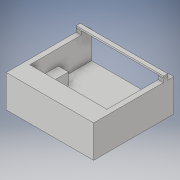
# Autodesk Inventor part: 0 - Ute
Saved by Autodesk Inventor 2019 (Build 230136000, 136)
## iProperties
Created: 2018-07-18
Part Number: 0 - Ute
Material: Generic
Document SubType Name: Modeling
Designer: Samuel
Density: 1 g/cm^3
Appearance: Default
Author: Samuel
Autodesk Inventor part; units mm, degrees
ref_plane "YZ Plane" through (0, 0, 0) normal (1, 0, 0) x (0, 1, 0)
ref_plane "XZ Plane" through (0, 0, 0) normal (0, 1, 0) x (-1, 0, 0)
ref_plane "XY Plane" through (0, 0, 0) normal (0, 0, 1) x (1, 0, 0)
sketch "Sketch1" plane through (0, 0, 0) normal (0, 1, 0) x (-1, 0, 0)
  line L0 (0, 0) -> (1500, 0)
  line L1 (1500, 0) -> (1500, -1460)
  line L2 (1500, -1460) -> (0, -1460)
  line L3 (0, -1460) -> (0, 0)
  dimension "d0" = 1500
  dimension "d1" = 1460
  constraints: 8 end point, 2 parallel, 1 horizontal, 1 perpendicular
  measures "d0" distance of L1.end L2.end
  measures "d1" distance of L0.end L1.end
extrude "Extrusion1" add sketch "Sketch1" against normal blind 100
sketch "Sketch2" plane through (0, 0, 0) normal (0, 1, 0) x (1, 0, 0)
  line L0 (-1500.0509, 0) -> (-1300.0509, 0)
  line L1 (-1300.0509, 0) -> (-1300.0509, 810)
  line L2 (-1300.0509, 810) -> (-1500.0509, 810)
  line L3 (-1500.0509, 810) -> (-1500.0509, 0)
  line L4 (0, 0) -> (-200, 0)
  line L5 (-200, 0) -> (-200, 810)
  line L6 (-200, 810) -> (0, 810)
  line L7 (0, 810) -> (0, 0)
  dimension "d4" = 200
  dimension "d5" = 810
  dimension "d6" = 200
  dimension "d7" = 810
  constraints: 16 end point, 4 parallel, 2 horizontal, 2 perpendicular
  measures "d4" distance of L2.end L1.end
  measures "d5" distance of L1.end L0.end
  measures "d6" distance of L5.end L6.end
  measures "d7" distance of L4.end L5.end
extrude "Extrusion2" add sketch "Sketch2" along normal blind 235
sketch "Sketch3" plane through (0, -100, 0) normal (0, -1, 0) x (1, 0, 0)
  line L0 (-1500, 0) -> (-1500, -1460) projected
  line L1 (0, 0) -> (-1500, 0)
  line L2 (-1500, 0) -> (-1500, -1460)
  line L3 (-1500, -1460) -> (0, -1460)
  line L4 (0, -1460) -> (0, 0)
  line L5 (-1500, -1460) -> (-1600, -1460)
  line L6 (-1600, -1460) -> (-1600, 0)
  line L7 (-1600, 0) -> (-1500, 0)
  line L8 (-1500, 0) -> (-1500, -1460)
  line L9 (0, -1460) -> (100, -1460)
  line L10 (100, -1460) -> (100, 0)
  line L11 (100, 0) -> (0, 0)
  line L12 (0, 0) -> (0, -1460)
  line L13 (100, 0) -> (-1600, 0)
  line L14 (-1600, 0) -> (-1600, 100)
  line L15 (-1600, 100) -> (100, 100)
  line L16 (100, 100) -> (100, 0)
  dimension "d10" = 100
  dimension "d11" = 100
  dimension "d12" = 1700
  dimension "d13" = 100
  constraints: 32 end point, 8 parallel, 4 horizontal, 4 perpendicular, 2 point on line
  measures "d10" distance of L6.end L7.end
  measures "d11" distance of L11.end L10.end
  measures "d12" distance of L14.end L15.end
  measures "d13" distance of L13.end L14.end
extrude "Extrusion3" add sketch "Sketch3" against normal blind 630 contours L7 L14 L15 L16 L11 L1 | L0 L5 L6 L7 | L11 L10 L9 L4
sketch "Sketch4" plane through (0, 0, -1460) normal (-1, 0, 0) x (0, 0, 1)
  line L0 (1460, 530) -> (1200, 530)
  line L1 (1200, 530) -> (1200, 470)
  line L2 (1200, 470) -> (1460, 470)
  line L3 (1460, 470) -> (1460, 530)
  point P0 (1460, 0)
  dimension "d16" = 260
  dimension "d17" = 60
  constraints: 8 end point, 2 parallel, 1 horizontal, 1 perpendicular
  measures "d16" distance of L2.end L1.end
  measures "d17" distance of L1.end L0.end
extrude "Extrusion4" add sketch "Sketch4" along normal blind 1500
sketch "Sketch5" plane through (0, 530, 0) normal (0, 1, 0) x (1, 0, 0)
  line L0 (100, 1460) -> (0, 1460) projected
  line L1 (100, -100) -> (100, 1460) projected
  line L2 (0, 1460) -> (100, 1460)
  line L3 (100, 1460) -> (100, 1340)
  line L4 (100, 1340) -> (0, 1340)
  line L5 (0, 1340) -> (0, 1460)
  line L6 (-1500, 1460) -> (-1600, 1460) projected
  line L7 (-1500, 260) -> (-1500, 1460) projected
  line L8 (-1600, 1460) -> (-1500, 1460)
  line L9 (-1500, 1460) -> (-1500, 1340)
  line L10 (-1500, 1340) -> (-1600, 1340)
  line L11 (-1600, 1340) -> (-1600, 1460)
  line L12 (0, 1340) -> (100, 1340)
  line L13 (100, 1340) -> (100, 1260)
  line L14 (100, 1260) -> (0, 1260)
  line L15 (0, 1260) -> (0, 1340)
  line L16 (-1600, 1460) -> (-1600, -100) projected
  line L17 (-1500, 1340) -> (-1600, 1340)
  line L18 (-1600, 1340) -> (-1600, 1260)
  line L19 (-1600, 1260) -> (-1500, 1260)
  line L20 (-1500, 1260) -> (-1500, 1340)
  point P0 (0, 0)
  dimension "d20" = 120
  dimension "d21" = 120
  dimension "d22" = 80
  dimension "d23" = 80
  constraints: 32 end point, 8 parallel, 4 horizontal, 4 perpendicular, 4 point on line
  measures "d20" distance of L2.end L3.end
  measures "d21" distance of L8.end L9.end
  measures "d22" distance of L12.end L13.end
  measures "d23" distance of L18.end L17.end
extrude "Extrusion5" add sketch "Sketch5" along normal blind 110 contours L1 L14 L15 L4 | L7 L19 L16 L10
sketch "Sketch6" plane through (100, 530, -1340) normal (0, 0, -1) x (-1, 0, 0)
  line L0 (0, 0) -> (0, 110) projected
  line L1 (100, 0) -> (100, 110) projected
  line L2 (0, 110) -> (100, 110)
  line L3 (100, 110) -> (100, 80)
  line L4 (100, 80) -> (0, 80)
  line L5 (0, 80) -> (0, 110)
  line L6 (0, 80) -> (1700, 80)
  line L7 (1700, 80) -> (1700, 60)
  line L8 (1700, 60) -> (0, 60)
  line L9 (0, 60) -> (0, 80)
  point P0 (100, -530)
  dimension "d26" = 30
  dimension "d27" = 1700
  dimension "d28" = 20
  constraints: 16 end point, 4 parallel, 2 horizontal, 2 perpendicular, 1 point on line
  measures "d26" distance of L2.end L3.end
  measures "d27" distance of L7.end L8.end
  measures "d28" distance of L6.end L7.end
extrude "Extrusion6" cut sketch "Sketch6" against normal blind 80 contours L0 L4 L1 L8 | L1 L6 L7 L8
sketch "Sketch7" plane through (0, 640, -1340) normal (-1, 0, 0) x (0, 0, 1)
  line L0 (80, -30) -> (80, 0) projected
  line L1 (0, 0) -> (80, 0)
  line L2 (80, 0) -> (80, -30)
  line L3 (80, -30) -> (0, -30)
  line L4 (0, -30) -> (0, 0)
  point P0 (1340, -640)
  dimension "d31" = 80
  dimension "d32" = 30
  constraints: 8 end point, 2 parallel, 1 horizontal, 1 perpendicular
  measures "d31" distance of L0.start L3.end
  measures "d32" distance of L1.end L0.start
extrude "Extrusion7" add sketch "Sketch7" along normal blind 1500
body "Solid1"
